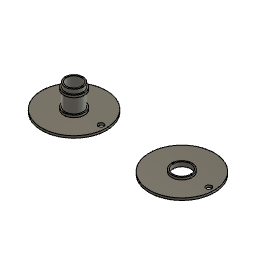
pickup bobbin fixed end v5 (Autodesk Fusion 360 design; units mm, degrees)
Autodesk Fusion 360 part; units mm, degrees
note: some values were not read from the file. Set by a fixed rule: which sketch regions a step uses.
sketch "main layout" plane through (0, 0, 0) normal (0, 1, 0) x (1, 0, 0)
  circle A0 centre (0, 0) radius 2.8
  circle A1 centre (0, 0) radius 3.3
  circle A2 centre (0, 0) radius 12
  line L0 (-3.5, 0) -> (3.5, 0)
  line L1 (0, 3.5) -> (0, -3)
  circle A3 centre (0, 0) radius 3.8
  circle A4 centre (10, -0.0014) radius 1
  dimension "d1" = 5.6
  dimension "d2" = 6.6
  dimension "d9" = 24
  dimension "d24" = 7.6
  dimension "d37" = 2
  dimension "d38" = 10
  constraint coincident A0.centre A1.centre
  constraint horizontal L0
  constraint vertical L1
  constraint concentric A0 A3
  measures "d1" diameter of A0
  measures "d2" diameter of A1
  measures "d9" diameter of A2
  measures "d24" diameter of A3
  measures "d37" diameter of A4
  measures "d38" distance of A0.centre A4.centre
extrude "Extrude2" add sketch "main layout" along normal blind 0.8 contours A2 | A3 | A4 makes body 1
extrude "Extrude1" add sketch "main layout" along normal blind 9.6 separate body contours A0 A1 L0 | A0 A1 L0 L1 | A0 A1 L0 L1 makes body 2
extrude "Extrude6" add sketch "main layout" against normal blind 0.8 from surface at 8 contours A3 bodies 2
extrude "Extrude5" add sketch "main layout" along normal blind 0.8 from surface at 0.8 contours A3 bodies 2
sketch "Sketch2" plane through (0, 9.6, 0) normal (0, 1, 0) x (-1, 0, 0)
  circle A0 centre (0, 0) radius 2.8
  circle A1 centre (0, 0) radius 3.3
  line L0 (0, 0) -> (-3.3, 0)
  line L1 (0, 0) -> (-1.65, -2.8579)
  line L2 (0, 0) -> (1.65, -2.8579)
  line L3 (0, 0) -> (3.3, 0)
  line L4 (0, 0) -> (1.65, 2.8579)
  line L5 (0, 0) -> (-1.65, 2.8579)
  dimension "d20" = 360
  constraint coincident A0.centre A1.centre
  constraint coincident A1 L0.end
  constraint horizontal L0
copy_body "CopyPasteBodies1" bodies 1 makes body 3
move_body "Move1" bodies 3 to x (1, 0, 0) y (0, 1, 0) z (0, 0, 1) at (40, 0, 0)
combine "Combine1" operation add target body 2 tool bodies 1
sketch "free end" plane through (0, 0.8, 0) normal (0, 1, 0) x (-1, 0, 0)
  circle A0 centre (-40, 0) radius 3.3
  circle A1 centre (-40, 0) radius 12
  circle A2 centre (-40, 0) radius 3.3
  circle A3 centre (-40, 0) radius 3.8
  circle A4 centre (-50, 0) radius 1
  dimension "d32" = 6.6
  dimension "d33" = 7.6
  dimension "d42" = 2
  dimension "d44" = 10
  measures "d32" diameter of A2
  measures "d33" diameter of A3
  measures "d42" diameter of A4
  measures "d44" distance of A0.centre A4.centre
extrude "Extrude7" add sketch "free end" along normal blind 0.8 contours A3 bodies 3
extrude "Extrude8" cut sketch "main layout" along normal blind 0.8 contours A4 bodies 2
extrude "Extrude9" cut sketch "free end" against normal blind 0.8 contours A4 bodies 3
equation "d1 = bore"
equation "d2 = bore + 2 * wallThickness"
equation "d3 = internalLength + 2 * endThickness"
equation "bore = 5.6 mm"
equation "wallThickness = 0.5 mm"
equation "endDia = 24 mm"
equation "endThickness = 0.8 mm"
equation "d9 = endDia"
equation "d10 = endThickness"
equation "internalLength = 8 mm"
equation "toothHeight = 0.5 mm"
equation "coreDia = bore + 2 * wallThickness"
equation "flangeDia = coreDia + 1 mm"
equation "d24 = flangeDia"
equation "d25 = endThickness"
equation "d26 = endThickness"
equation "d28 = internalLength + endThickness - endThickness"
equation "d29 = -endThickness"
equation "d32 = bore + 2 * wallThickness"
equation "d33 = flangeDia"
equation "d34 = endThickness"
equation "wireHoleDia = 2 mm"
equation "d37 = wireHoleDia"
equation "d38 = wireHolePos"
equation "d39 = endThickness"
equation "d42 = wireHoleDia"
equation "wireHolePos = endDia / 2 - wireHoleDia / 2 - 1 mm"
equation "d44 = wireHolePos"
equation "d45 = -endThickness"
named bodies: "end", "core"
